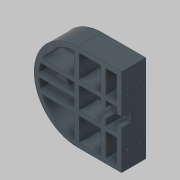
# Autodesk Inventor part: NA001
Saved by Autodesk Inventor 2017 (Build 210142000, 142)
## iProperties
Created: 2017-06-04
Part Number: NA001
Material: ABS Plastic
Document SubType Name: Modeling
Designer: Zach
Density: 1.06 g/cm^3
Appearance: CR Dark Blue
Author: Zach
Autodesk Inventor part; units mm, degrees
ref_plane "YZ Plane" through (0, 0, 0) normal (1, 0, 0) x (0, 1, 0)
ref_plane "XZ Plane" through (0, 0, 0) normal (0, 1, 0) x (-1, 0, 0)
ref_plane "XY Plane" through (0, 0, 0) normal (0, 0, 1) x (1, 0, 0)
sketch "Sketch1" plane through (0, 0, 0) normal (0, 0, 1) x (1, 0, 0)
  line L0 (0, 0) -> (180, 0)
  line L1 (180, 0) -> (180, 180)
  line L2 (180, 180) -> (0, 180)
  line L3 (0, 180) -> (0, 0)
  circle A0 centre (50, 90) radius 6
  point P0 (180, 90)
  dimension "d0" = 180
  dimension "d1" = 180
  dimension "d2" = 12
  dimension "d7" = 50
  constraints: 8 end point, 2 parallel, 1 centre point, 1 horizontal, 1 horizontal alignment, 1 midpoint, 1 perpendicular
  measures "d0" distance of L2.end L1.end
  measures "d1" distance of L1.end L0.end
  measures "d2" diameter of A0
  measures "d7" distance from line of L3 A0.centre
extrude "Extrusion1" add sketch "Sketch1" along normal blind 10
sketch "Sketch2" plane through (0, 0, 10) normal (0, 0, 1) x (1, 0, 0)
  circle A0 centre (115, 90) radius 3
  line L0 (180, 0) -> (180, 180) projected
  circle A1 centre (50, 90) radius 6 projected
  line L1 (0, 0) -> (180, 0) projected
  line L2 (180, 0) -> (180, 180) projected
  line L3 (180, 180) -> (0, 180) projected
  line L4 (0, 180) -> (0, 0) projected
  point P0 (180, 90)
  dimension "d8" = 6
  dimension "d9" = 65
  constraints: 1 centre point, 1 horizontal alignment, 1 midpoint
  measures "d8" diameter of A0
  measures "d9" distance of A0.centre A1.centre
extrude "Extrusion2" cut sketch "Sketch2" against normal through all contours A0
sketch "Sketch3" plane through (0, 0, 10) normal (0, 0, 1) x (1, 0, 0)
  circle A0 centre (115, 90) radius 3 construction
  circle A1 centre (50, 90) radius 6 projected
  line L0 (0, 0) -> (180, 0) projected
  line L1 (180, 0) -> (180, 180) projected
  line L2 (180, 180) -> (0, 180) projected
  line L3 (0, 180) -> (0, 0) projected
  line L4 (99.5, 74.5) -> (130.5, 74.5) construction
  line L5 (130.5, 74.5) -> (130.5, 105.5) construction
  line L6 (130.5, 105.5) -> (99.5, 105.5) construction
  line L7 (99.5, 105.5) -> (99.5, 74.5) construction
  line L8 (99.5, 74.5) -> (130.5, 105.5) construction
  line L9 (130.5, 74.5) -> (99.5, 105.5) construction
  circle A2 centre (99.5, 105.5) radius 1.65
  circle A3 centre (130.5, 105.5) radius 1.65
  circle A4 centre (130.5, 74.5) radius 1.65
  circle A5 centre (99.5, 74.5) radius 1.65
  dimension "d12" = 31
  dimension "d13" = 31
  dimension "d14" = 3.3
  dimension "d15" = 3.3
  dimension "d16" = 3.3
  dimension "d17" = 3.3
  constraints: 12 end point, 4 centre point, 4 coincident, 2 midpoint, 2 parallel, 1 horizontal, 1 perpendicular
  measures "d12" distance of L6.end L5.end
  measures "d13" distance of L5.end L4.end
  measures "d14" diameter of A2
  measures "d15" diameter of A3
  measures "d16" diameter of A4
  measures "d17" diameter of A5
extrude "Extrusion3" cut sketch "Sketch3" against normal through all contours A2 | A3 | A4 | A5
sketch "Sketch4" plane through (0, 0, 10) normal (0, 0, 1) x (1, 0, 0)
  circle A0 centre (130.5, 74.5) radius 1.65 projected
  circle A1 centre (99.5, 105.5) radius 1.65 projected
  circle A2 centre (130.5, 105.5) radius 1.65 projected
  circle A3 centre (99.5, 74.5) radius 1.65 projected
  circle A4 centre (115, 90) radius 3 projected
  circle A5 centre (50, 90) radius 6 projected
  line L0 (0, 0) -> (180, 0) projected
  line L1 (180, 0) -> (180, 180) projected
  line L2 (180, 180) -> (0, 180) projected
  line L3 (0, 180) -> (0, 0) projected
  circle A6 centre (115, 90) radius 12.5
  dimension "d20" = 25
  constraints: 1 centre point, 1 coincident
  measures "d20" diameter of A6
extrude "Extrusion4" cut sketch "Sketch4" against normal blind 2 contours A6
sketch "Sketch5" plane through (0, 0, 10) normal (0, 0, 1) x (1, 0, 0)
  circle A0 centre (115, 90) radius 12.5 projected
  circle A1 centre (130.5, 74.5) radius 1.65 projected
  circle A2 centre (99.5, 105.5) radius 1.65 projected
  circle A3 centre (130.5, 105.5) radius 1.65 projected
  circle A4 centre (99.5, 74.5) radius 1.65 projected
  circle A5 centre (50, 90) radius 6 projected
  line L0 (0, 0) -> (180, 0) projected
  line L1 (180, 0) -> (180, 180) projected
  line L2 (180, 180) -> (0, 180) projected
  line L3 (0, 180) -> (0, 0) projected
  circle A6 centre (90, 90) radius 90 construction
  line L4 (0, 0) -> (180, 0) projected
  arc A7 (90, 180) -> (90, 0) centre (90, 90) ccw
  line L5 (180, 180) -> (0, 180) projected
  line L6 (90, 180) -> (0, 180)
  line L7 (0, 180) -> (0, 0)
  line L8 (90, 0) -> (0, 0)
  point P0 (0, 90)
  constraints: 6 end point, 4 point on circle, 4 tangent, 3 midpoint, 2 centre point, 2 collinear, 1 horizontal alignment, 1 perpendicular
extrude "Extrusion5" cut sketch "Sketch5" against normal through all contours L3 A7 L0 | L3 L2 A7
sketch "Sketch6" plane through (0, 0, 10) normal (0, 0, 1) x (1, 0, 0)
  circle A0 centre (99.5, 74.5) radius 1.65 projected
  circle A1 centre (130.5, 105.5) radius 1.65 projected
  circle A2 centre (99.5, 105.5) radius 1.65 projected
  circle A3 centre (130.5, 74.5) radius 1.65 projected
  circle A4 centre (115, 90) radius 12.5 projected
  arc A5 (90, 180) -> (90, 0) centre (90, 90) ccw projected
  line L0 (90, 0) -> (180, 0) projected
  line L1 (180, 0) -> (180, 180) projected
  line L2 (180, 180) -> (90, 180) projected
  circle A6 centre (50, 90) radius 6
  circle A7 centre (50, 90) radius 16
  point P0 (0, 0)
  dimension "d25" = 12
  dimension "d26" = 32
  constraints: 8 centre point, 1 coincident
  measures "d25" diameter of A6
  measures "d26" diameter of A7
extrude "Extrusion6" add sketch "Sketch6" along normal blind 27.5 contours A7
sketch "Sketch7" plane through (50, 90, 37.5) normal (0, 0, 1) x (1, 0, 0)
  circle A0 centre (0, 0) radius 16
  point P0 (-50, -90)
  constraints: 1 centre point
extrude "Extrusion7" add sketch "Sketch7" along normal blind 5
sketch "Sketch8" plane through (0, 0, 10) normal (0, 0, 1) x (1, 0, 0)
  circle A0 centre (50, 90) radius 16 projected
  circle A1 centre (99.5, 74.5) radius 1.65 projected
  circle A2 centre (130.5, 105.5) radius 1.65 projected
  circle A3 centre (99.5, 105.5) radius 1.65 projected
  circle A4 centre (130.5, 74.5) radius 1.65 projected
  circle A5 centre (115, 90) radius 12.5 projected
  arc A6 (90, 180) -> (90, 0) centre (90, 90) ccw projected
  line L0 (90, 0) -> (180, 0) projected
  line L1 (180, 0) -> (180, 180) projected
  line L2 (180, 180) -> (90, 180) projected
  line L3 (92.5, 67.5) -> (137.5, 67.5)
  line L4 (137.5, 67.5) -> (137.5, 112.5)
  line L5 (137.5, 112.5) -> (92.5, 112.5)
  line L6 (92.5, 112.5) -> (92.5, 67.5)
  circle A7 centre (115, 90) radius 3 projected
  line L7 (92.5, 67.5) -> (137.5, 112.5) construction
  line L8 (137.5, 67.5) -> (92.5, 112.5) construction
  arc A8 (90, 170) -> (90, 10) centre (90, 90) ccw
  line L9 (90, 170) -> (170, 170)
  line L10 (170, 170) -> (170, 10)
  line L11 (170, 10) -> (90, 10)
  line L12 (82.5, 57.5) -> (147.5, 57.5)
  line L13 (147.5, 57.5) -> (147.5, 122.5)
  line L14 (147.5, 122.5) -> (82.5, 122.5)
  line L15 (82.5, 122.5) -> (82.5, 57.5)
  point P0 (0, 0)
  dimension "d32" = 45
  dimension "d33" = 45
  dimension "d34" = 10
  dimension "d35" = 10
  constraints: 26 end point, 4 parallel, 2 midpoint, 2 perpendicular, 2 point on circle, 1 centre point, 1 horizontal, 6 other
  measures "d32" distance of L5.end L4.end
  measures "d33" distance of L4.end L3.end
  measures "d34" radial gap between concentric circles of A6 A8
  measures "d35" distance between parallel lines of L6 L15
extrude "Extrusion8" add sketch "Sketch8" along normal blind 40 contours L2 L1 L0 A6 | L15 L14 L13 L12
sketch "Sketch9" plane through (0, 0, 10) normal (0, 0, 1) x (1, 0, 0)
  circle A0 centre (50, 90) radius 16 projected
  line L0 (170, 170) -> (90, 170) projected
  arc A1 (90, 170) -> (90, 10) centre (90, 90) ccw projected
  line L1 (90, 10) -> (170, 10) projected
  line L2 (170, 10) -> (170, 170) projected
  line L3 (82.5, 57.5) -> (82.5, 122.5) projected
  line L4 (82.5, 122.5) -> (147.5, 122.5) projected
  line L5 (147.5, 122.5) -> (147.5, 57.5) projected
  line L6 (147.5, 57.5) -> (82.5, 57.5) projected
  line L7 (147.5, 85) -> (170, 85)
  line L8 (147.5, 95) -> (170, 95)
  line L9 (147.5, 90) -> (170, 90) construction
  line L10 (147.5, 95) -> (147.5, 85)
  line L11 (170, 95) -> (170, 85)
  line L12 (147.5, 57.5) -> (170, 57.5)
  line L13 (147.5, 67.5) -> (170, 67.5)
  line L14 (147.5, 67.5) -> (147.5, 57.5)
  line L15 (170, 67.5) -> (170, 57.5)
  line L16 (147.5, 122.5) -> (170, 122.5)
  line L17 (147.5, 112.5) -> (170, 112.5)
  line L18 (170, 112.5) -> (170, 122.5)
  line L19 (147.5, 122.5) -> (147.5, 112.5)
  line L20 (82.5, 57.5) -> (82.5, 122.5) projected
  line L21 (82.5, 122.5) -> (16.899, 122.5)
  arc A2 (90, 170) -> (90, 10) centre (90, 90) ccw projected
  line L22 (82.5, 112.5) -> (13.2292, 112.5)
  line L23 (82.5, 57.5) -> (147.5, 57.5) projected
  line L24 (82.5, 57.5) -> (16.899, 57.5)
  line L25 (82.5, 67.5) -> (13.2292, 67.5)
  line L26 (82.5, 85) -> (10.1564, 85)
  line L27 (82.5, 95) -> (10.1564, 95)
  arc A3 (16.899, 122.5) -> (13.2292, 112.5) centre (90, 90) ccw
  arc A4 (10.1564, 95) -> (10.1564, 85) centre (90, 90) ccw
  arc A5 (13.2292, 67.5) -> (16.899, 57.5) centre (90, 90) ccw
  line L28 (82.5, 122.5) -> (82.5, 112.5)
  line L29 (82.5, 95) -> (82.5, 85)
  line L30 (82.5, 67.5) -> (82.5, 57.5)
  line L31 (82.5, 122.5) -> (147.5, 122.5) projected
  line L32 (82.5, 122.5) -> (82.5, 169.6477)
  line L33 (147.5, 57.5) -> (82.5, 57.5) projected
  line L34 (82.5, 57.5) -> (82.5, 10.3523)
  line L35 (92.5, 122.5) -> (92.5, 170)
  line L36 (92.5, 57.5) -> (92.5, 10)
  arc A6 (92.5, 170) -> (82.5, 169.6477) centre (89.0747, 125.1306) ccw
  arc A7 (82.5, 10.3523) -> (92.5, 10) centre (89.0747, 54.8694) ccw
  line L37 (82.5, 122.5) -> (92.5, 122.5)
  line L38 (82.5, 57.5) -> (92.5, 57.5)
  line L39 (147.5, 122.5) -> (147.5, 170)
  line L40 (170, 170) -> (90, 170) projected
  line L41 (137.5, 122.5) -> (137.5, 170)
  line L42 (147.5, 57.5) -> (147.5, 10)
  line L43 (90, 10) -> (170, 10) projected
  line L44 (137.5, 57.5) -> (137.5, 10)
  line L45 (137.5, 57.5) -> (147.5, 57.5)
  line L46 (147.5, 10) -> (137.5, 10)
  line L47 (137.5, 170) -> (147.5, 170)
  line L48 (137.5, 122.5) -> (147.5, 122.5)
  point P0 (0, 0)
  dimension "d38" = 10
  dimension "d39" = 10
  dimension "d40" = 10
  dimension "d43" = 10
  dimension "d44" = 10
  dimension "d45" = 10
  dimension "d46" = 45
  dimension "d47" = 45
  constraints: 72 end point, 22 point on line, 10 point on circle, 9 collinear, 7 horizontal, 7 perpendicular, 6 vertical, 5 centre point, 4 horizontal alignment, 3 parallel, 1 midpoint, 18 other
  measures "d38" distance between parallel lines of L7 L8
  measures "d39" distance between parallel lines of L13 L12
  measures "d40" distance between parallel lines of L16 L17
  measures "d43" distance between parallel lines of L36 L34
  measures "d44" distance between parallel lines of L35 L32
  measures "d45" distance between parallel lines of L39 L41
  measures "d46" radius of A6
  measures "d47" radius of A7
extrude "Extrusion9" add sketch "Sketch9" along normal blind 40 contours A0 L26 L27 | A0 L27 L3 L26 | A0 L26 A1 L27 | L22 A1 L21 L3 | L3 L24 A1 L25 | L32 A1 L0 L35 L4 | L6 L36 L1 A1 L34 | A6 L0 A1 | L41 L0 L39 L4 | L6 L42 L1 L44 | L16 L2 L17 L5 | L5 L13 L2 L12 | L8 L2 L7 L5
sketch "Sketch10" plane through (0, 0, 50) normal (0, 0, 1) x (1, 0, 0)
  line L0 (137.5, 100) -> (180, 100)
  line L1 (180, 100) -> (180, 80)
  line L2 (180, 80) -> (137.5, 80)
  line L3 (137.5, 80) -> (137.5, 100)
  line L4 (137.5, 112.5) -> (137.5, 67.5) projected
  circle A0 centre (115, 90) radius 3 construction
  line L5 (115, 90) -> (193.2045, 90) construction
  line L6 (180, 0) -> (180, 180) projected
  point P0 (0, 0)
  dimension "d48" = 20
  constraints: 10 end point, 2 horizontal, 2 parallel, 2 point on line, 1 perpendicular, 1 other
  measures "d48" distance between parallel lines of L2 L0
extrude "Extrusion10" cut sketch "Sketch10" against normal blind 20
sketch "Sketch11" plane through (180, 0, 0) normal (1, 0, 0) x (0, 0, -1)
  circle A0 centre (-37.5, 35) radius 2.5
  circle A1 centre (-12.5, 35) radius 2.5
  circle A2 centre (-37.5, 145) radius 2.5
  circle A3 centre (-12.5, 145) radius 2.5
  line L0 (0, 0) -> (-50, 0) projected
  line L1 (-50, 0) -> (-50, 80) projected
  line L2 (0, 180) -> (-50, 180) projected
  dimension "d51" = 5
  dimension "d52" = 5
  dimension "d53" = 5
  dimension "d54" = 5
  dimension "d55" = 35
  dimension "d56" = 12.5
  dimension "d57" = 25
  dimension "d58" = 35
  constraints: 4 centre point, 2 horizontal alignment, 2 vertical alignment
  measures "d51" diameter of A0
  measures "d52" diameter of A1
  measures "d53" diameter of A2
  measures "d54" diameter of A3
  measures "d55" distance from line of L0 A0.centre
  measures "d56" distance from line of A0.centre L1
  measures "d57" distance of A0.centre A1.centre
  measures "d58" distance from line of L2 A2.centre
extrude "Extrusion11" cut sketch "Sketch11" against normal blind 10
sketch "Sketch12" plane through (0, 0, 0) normal (0, 0, -1) x (-1, 0, 0)
  circle A0 centre (-50, 90) radius 6
  arc A1 (-90, 0) -> (-90, 180) centre (-90, 90) ccw projected
  line L0 (-180, 180) -> (-90, 180) projected
  line L1 (-180, 0) -> (-180, 180) projected
  line L2 (-90, 0) -> (-180, 0) projected
  circle A2 centre (-130.5, 74.5) radius 1.65 projected
  circle A3 centre (-99.5, 105.5) radius 1.65 projected
  circle A4 centre (-130.5, 105.5) radius 1.65 projected
  circle A5 centre (-99.5, 74.5) radius 1.65 projected
  circle A6 centre (-115, 90) radius 3 projected
  circle A7 centre (-50, 90) radius 6 projected
  circle A8 centre (-50, 90) radius 6 projected
  point P0 (0, 0)
  dimension "d61" = 12
  constraints: 1 centre point, 1 concentric
  measures "d61" diameter of A0
extrude "Extrusion12" cut sketch "Sketch12" against normal blind 37.5 contours A0
body "Solid1"
